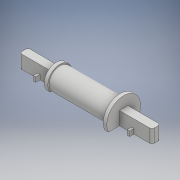
# Autodesk Inventor part: mini
Saved by Autodesk Inventor 2018 (Build 220112000, 112)
## iProperties
Created: 2018-09-11
Part Number: mini
Material: Generic
Document SubType Name: Modeling
Designer: erwin
Density: 1 g/cm^3
Appearance: Default
Author: erwin
Autodesk Inventor part; units mm, degrees
ref_plane "YZ Plane" through (0, 0, 0) normal (1, 0, 0) x (0, 1, 0)
ref_plane "XZ Plane" through (0, 0, 0) normal (0, 1, 0) x (-1, 0, 0)
ref_plane "XY Plane" through (0, 0, 0) normal (0, 0, 1) x (1, 0, 0)
sketch "Sketch1" plane through (0, 0, 0) normal (1, 0, 0) x (0, 1, 0)
  circle A0 centre (0, 0) radius 10 construction
  line L0 (3.5, 5) -> (-3.5, 5)
  line L1 (-3.5, 5) -> (-3.5, -5)
  line L2 (-3.5, -5) -> (3.5, -5)
  line L3 (3.5, -5) -> (3.5, 5)
  line L4 (3.5, 5) -> (-3.5, -5) construction
  line L5 (-3.5, 5) -> (3.5, -5) construction
  dimension "d0" = 20
  dimension "d1" = 7
  dimension "d2" = 10
  constraints: 12 end point, 2 midpoint, 2 parallel, 1 centre point, 1 coincident, 1 horizontal, 1 perpendicular
  measures "d0" diameter of A0
  measures "d1" distance of L2.end L1.end
  measures "d2" distance of L1.end L0.end
extrude "Extrusion1" add sketch "Sketch1" along normal blind 110
ref_plane "Work Plane1" through (55, 0, 0) normal (-1, 0, 0) x (0, 0, 1)
sketch "Sketch2" plane through (55, 0, 0) normal (-1, 0, 0) x (0, 0, 1)
  arc A0 (-6, -6.7082) -> (-6, 6.7082) centre (0, 0) ccw
  line L0 (-5, -3.5) -> (-5, 3.5) projected
  line L1 (-6, -6.7082) -> (-6, 6.7082)
  dimension "d5" = 18
  constraints: 2 end point, 2 point on circle, 1 centre point, 1 coincident, 1 parallel
  measures "d5" diameter of A0
extrude "Extrusion2" add sketch "Sketch2" along normal mid plane 50
sketch "Sketch3" plane through (80, 0, 0) normal (1, 0, 0) x (0, 0, -1)
  arc A0 (6, 6.7082) -> (6, -6.7082) centre (0, 0) ccw projected
  arc A1 (6, 12.6491) -> (6, -12.6491) centre (0, 0) ccw
  line L0 (6, 6.7082) -> (6, -6.7082) projected
  line L1 (6, 12.6491) -> (6, -12.6491)
  dimension "d8" = 5
  constraints: 2 end point, 2 point on circle, 1 centre point, 1 collinear
  measures "d8" radial gap between concentric circles of A0 A1
extrude "Extrusion3" add sketch "Sketch3" along normal blind 3
mirror "Mirror1" about plane through (55, 0, 0) normal (-1, 0, 0) of "Extrusion3"
thicken "Thicken1" operation add thickness 4 both sides no extend neighbours yes toward (0, 0.6817885, -0.7315493) faces at (28, -9.545, 10.2417)
fillet "Fillet1" radius 2 4 edges at (110, -3.5, 0) (110, 3.5, 0) (0, -3.5, 0) (0, 3.5, 0)
move faces "Move1" translate (0, 0, -1) faces at (91.3333, -1.1667, -5) (10.3333, -1.1667, -5)
sketch "Sketch4" plane through (27, -3.5, -6) normal (0, 0, 1) x (1, 0, 0)
  line L0 (3, 10.2082) -> (53, 10.2082) projected
  line L1 (3, -3.2082) -> (3, 10.2082) projected
  line L2 (53, -3.2082) -> (3, -3.2082) projected
  line L3 (53, 10.2082) -> (53, -3.2082) projected
  line L4 (68, -3.5) -> (-12, -3.5)
  line L5 (-12, -3.5) -> (-12, 10.5)
  line L6 (-12, 10.5) -> (68, 10.5)
  line L7 (68, 10.5) -> (68, -3.5)
  line L8 (68, -3.5) -> (-12, 10.5) construction
  line L9 (-12, -3.5) -> (68, 10.5) construction
  line L10 (-12, -3.5) -> (-10, -3.5)
  line L11 (-10, -3.5) -> (-10, 10.15)
  line L12 (-10, 10.15) -> (-12, 10.15)
  line L13 (-12, 10.15) -> (-12, -3.5)
  point P0 (-27, 3.5)
  point P1 (28, 3.5)
  dimension "d18" = 80
  dimension "d19" = 14
  dimension "d20" = 2
  constraints: 20 end point, 4 parallel, 2 horizontal, 2 midpoint, 2 perpendicular, 1 point on line
  measures "d18" distance of L5.end L6.end
  measures "d19" distance of L4.end L5.end
  measures "d20" distance of L12.end L11.end
extrude "Extrusion4" add sketch "Sketch4" along normal blind 4 contours L4 L5 L12 L11
mirror "Mirror2" about plane through (55, 0, 0) normal (-1, 0, 0) of "Extrusion4"
body "Solid1"
